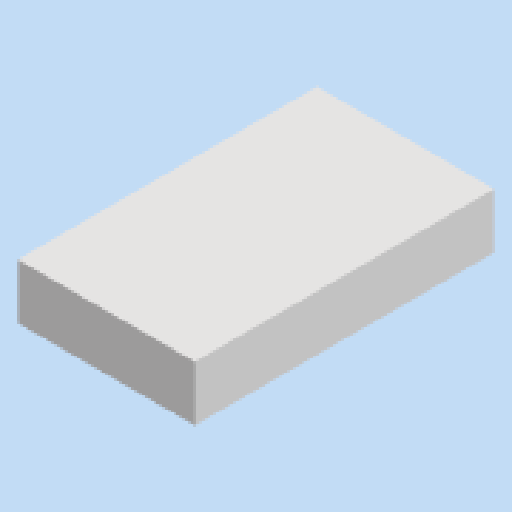
# Autodesk Inventor part: pegshort
Saved by Autodesk Inventor 2023 (Build 270158000, 158)
## iProperties
Created: 2026-03-30
Part Number: pegshort
Material: Generic
Document SubType Name: Modeling
Designer: Nathann
Density: 1 g/cm^3
Appearance: Default
Author: Nathann
Autodesk Inventor part; units mm, degrees
ref_plane "YZ Plane" through (0, 0, 0) normal (1, 0, 0) x (0, 1, 0)
ref_plane "XZ Plane" through (0, 0, 0) normal (0, 1, 0) x (-1, 0, 0)
ref_plane "XY Plane" through (0, 0, 0) normal (0, 0, 1) x (1, 0, 0)
sketch "Sketch1" plane through (0, 0, 0) normal (0, 1, 0) x (-1, 0, 0)
  line L0 (0, 0) -> (29, 0)
  line L1 (29, 0) -> (29, 49)
  line L2 (29, 49) -> (0, 49)
  line L3 (0, 49) -> (0, 0)
  dimension "d0" = 49
  dimension "d1" = 29
  constraints: 8 end point, 2 parallel, 1 horizontal, 1 perpendicular
  measures "d0" distance of L0.end L1.end
  measures "d1" distance of L1.end L2.end
extrude "Extrusion1" add sketch "Sketch1" along normal blind 9
sketch "Sketch2" plane through (0, 0, 0) normal (0, -1, 0) x (1, 0, 0)
  line L0 (-21.7451, 36.3583) -> (64.7541, 36.3583) construction
  line L1 (64.7541, 36.3583) -> (64.7541, 15.5155) construction
  line L2 (64.7541, 15.5155) -> (-21.7451, 15.5155) construction
  line L3 (-21.7451, 15.5155) -> (-21.7451, 36.3583) construction
  spline S0 degree 2 poles (-14.1438, 15.6452) (-16.3156, 15.6452) (-19.3626, 16.5528) (-20.7078, 17.2011) knots 0 0 0 1 2 2 2
  line L4 (-20.7078, 17.2011) -> (-20.7078, 20.5398)
  line L5 (-20.7078, 20.5398) -> (-20.5133, 20.5398)
  spline S1 degree 2 poles (-20.5133, 20.5398) (-19.2005, 19.3081) (-15.878, 17.9466) (-14.3383, 17.9466) knots 0 0 0 1 2 2 2
  spline S2 degree 2 poles (-14.3383, 17.9466) (-12.134, 17.9466) (-9.8812, 19.7781) (-9.8812, 21.2854) knots 0 0 0 1 2 2 2
  spline S3 degree 2 poles (-9.8812, 21.2854) (-9.8812, 22.4847) (-11.0644, 23.9758) (-12.3447, 24.3486) knots 0 0 0 1 2 2 2
  spline S4 degree 2 poles (-12.3447, 24.3486) (-13.2686, 24.6079) (-14.8083, 24.9645) (-15.959, 25.2562) knots 0 0 0 1 2 2 2
  spline S5 degree 2 poles (-15.959, 25.2562) (-16.9963, 25.5317) (-18.6332, 26.3583) (-19.2653, 27.0228) knots 0 0 0 1 2 2 2
  spline S6 degree 2 poles (-19.2653, 27.0228) (-19.8812, 27.6873) (-20.5619, 29.4701) (-20.5619, 30.6371) knots 0 0 0 1 2 2 2
  spline S7 degree 2 poles (-20.5619, 30.6371) (-20.5619, 33.0682) (-16.7694, 36.3583) (-13.8358, 36.3583) knots 0 0 0 1 2 2 2
  spline S8 degree 2 poles (-13.8358, 36.3583) (-12.1503, 36.3583) (-9.1681, 35.6938) (-7.8877, 35.0617) knots 0 0 0 1 2 2 2
  line L6 (-7.8877, 35.0617) -> (-7.8877, 31.8851)
  line L7 (-7.8877, 31.8851) -> (-8.0822, 31.8851)
  spline S9 degree 2 poles (-8.0822, 31.8851) (-9.0384, 32.7603) (-12.0206, 34.0569) (-13.6575, 34.0569) knots 0 0 0 1 2 2 2
  spline S10 degree 2 poles (-13.6575, 34.0569) (-15.5052, 34.0569) (-17.7904, 32.3227) (-17.7904, 30.9126) knots 0 0 0 1 2 2 2
  spline S11 degree 2 poles (-17.7904, 30.9126) (-17.7904, 29.6484) (-16.4452, 28.1411) (-15.181, 27.8008) knots 0 0 0 1 2 2 2
  spline S12 degree 2 poles (-15.181, 27.8008) (-14.3383, 27.5739) (-11.8909, 26.9904) (-11.0806, 26.7473) knots 0 0 0 1 2 2 2
  spline S13 degree 2 poles (-11.0806, 26.7473) (-9.0222, 26.1152) (-7.1097, 23.5706) (-7.1097, 21.7068) knots 0 0 0 1 2 2 2
  spline S14 degree 2 poles (-7.1097, 21.7068) (-7.1097, 20.5236) (-8.066, 18.2546) (-8.925, 17.4604) knots 0 0 0 1 2 2 2
  spline S15 degree 2 poles (-8.925, 17.4604) (-9.8812, 16.5852) (-12.3123, 15.6452) (-14.1438, 15.6452) knots 0 0 0 1 2 2 2
  point P0 (0, 0)
  constraints: 2 other
emboss "Emboss1" sketch "Sketch2" operation cut depth 2 direction (0, 1, 0)
body "Solid1"
